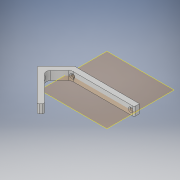
# Autodesk Inventor part: Part5
Saved by Autodesk Inventor 2019 (Build 230136000, 136)
## iProperties
Created: 2021-11-18
Part Number: Part5
Material: Generic
Document SubType Name: Modeling
Designer: Pokick
Density: 1 g/cm^3
Appearance: Default
Author: Pokick
Autodesk Inventor part; units mm, degrees
ref_plane "YZ Plane" through (0, 0, 0) normal (1, 0, 0) x (0, 1, 0)
ref_plane "XY Plane" through (0, 0, 0) normal (0, 0, 1) x (1, 0, 0)
sketch "Sketch1" plane through (0, 0, 0) normal (0, 0, 1) x (1, 0, 0)
  line L0 (-33, 45) -> (33, 45) construction
  line L1 (33, 45) -> (33, -45) construction
  line L2 (33, -45) -> (-33, -45) construction
  line L3 (-33, -45) -> (-33, 45) construction
  line L4 (-33, 45) -> (33, -45) construction
  line L5 (33, 45) -> (-33, -45) construction
  circle A0 centre (33, 45) radius 1.7
  circle A1 centre (-33, 45) radius 1.7
  point P0 (0, 0)
  dimension "d0" = 66
  dimension "d1" = 90
  dimension "d2" = 3.4
  dimension "d3" = 3.4
  constraints: 12 end point, 2 centre point, 2 coincident, 2 midpoint, 2 parallel, 1 horizontal, 1 perpendicular
  measures "d0" distance of L1.end L2.end
  measures "d1" distance of L0.end L1.end
  measures "d2" diameter of A0
  measures "d3" diameter of A1
ref_plane "Work Plane1" through (0, 45, 0) normal (0, 1, 0) x (-1, 0, 0)
sketch "Sketch2" plane through (0, 45, 0) normal (0, 1, 0) x (-1, 0, 0)
  line L0 (0, 0) -> (-37, 0)
  line L1 (0, 0) -> (37, 0)
  line L2 (37, 0) -> (58.2132, 21.2132)
  line L3 (58.2132, 21.2132) -> (-12.4975, 91.9239) construction
  line L4 (58.2132, 21.2132) -> (158.2132, 21.2132) construction
  line L5 (-37, 0) -> (21.2132, 58.2132) construction
  line L6 (-37, 0) -> (45.3259, 0) construction
  line L7 (21.2132, 58.2132) -> (58.2132, 21.2132)
  line L8 (37, 0) -> (37, 6) construction
  line L9 (43.7619, 6.7619) -> (39.5192, 11.0045) construction
  line L10 (43.7619, 6.7619) -> (49.7619, 6.7619) construction
  line L11 (34.5147, 6) -> (-31, 6)
  line L12 (-31, 6) -> (-37, 0) construction
  line L13 (39.5192, 11.0045) -> (34.5147, 6)
  line L14 (53.9706, 25.4558) -> (49.7279, 21.2132) construction
  line L15 (39.5192, 11.0045) -> (49.7279, 21.2132)
  line L16 (21.2132, 58.2132) -> (16.9706, 53.9706)
  line L17 (49.7279, 21.2132) -> (16.9706, 53.9706)
  line L18 (-37, 0) -> (-37, 6)
  line L19 (-37, 6) -> (-31, 6)
  dimension "d5" = 37
  dimension "d6" = 37
  dimension "d7" = 30
  dimension "d8" = 135
  dimension "d9" = 100
  dimension "d10" = 135
  dimension "d11" = 45
  dimension "d13" = 6
  dimension "d14" = 6
  dimension "d15" = 135
  dimension "d16" = 14.4513
  dimension "d17" = 6
  dimension "d18" = 20.1629
  dimension "d19" = 15.2132
  constraints: 40 end point, 6 horizontal, 5 point on line, 3 equal length, 3 perpendicular, 2 collinear, 2 vertical, 1 parallel
  measures "d5" distance of L0.start L0.end
  measures "d6" distance of L0.start L1.end
  measures "d7" distance of L1.end L2.end
  measures "d8" angle of L2 L1
  measures "d9" distance of L2.end L3.end
  measures "d10" angle of L4 L3
  measures "d11" angle of L6 L5
  measures "d13" distance of L1.end L8.end
  measures "d14" distance of L9.start L9.end
  measures "d15" angle of L10 L9
  measures "d16" distance between parallel lines of L10 L4
  measures "d17" distance of L14.start L14.end
  measures "d18" distance from line of L0.start L14
  measures "d19" distance between parallel lines of L11 L4
extrude "Extrusion1" add sketch "Sketch2" along normal mid plane 10
fillet "Fillet1" radius 5 2 edges at (-49.7279, 45, 21.2132) (-34.5147, 45, 6)
fillet "Fillet2" radius 0.5 1 edges at (37, 45, 0)
fillet "Fillet3" radius 2 1 edges at (-37, 45, 0)
fillet "Fillet4" radius 2 3 edges at (-58.2132, 45, 21.2132) (-16.9706, 45, 53.9706) (-21.2132, 45, 58.2132)
fillet "Fillet5" radius 2 1 edges at (37, 45, 6)
extrude "Extrusion2" cut sketch "Sketch1" along normal blind 10
sketch "Sketch3" plane through (-22.6274, 40, 56.799) normal (-0.7071068, 0, 0.7071068) x (0.7071068, 0, 0.7071068)
  line L0 (-39.3259, 0) -> (0, 0) construction
  line L1 (-48.3259, 0) -> (-48.3259, 10) construction
  line L2 (0, 0) -> (-48.3259, 0) construction
  line L3 (-48.3259, 0) -> (-48.3259, 10) construction
  line L4 (-48.3259, 10) -> (0, 10) construction
  line L5 (0, 10) -> (0, 0) construction
  line L6 (0, 0) -> (0, 10) projected
  line L7 (0, 5) -> (-48.6996, 5) construction
  ellipse E0 centre (-47.4975, 5) end of major axis (-47.4975, 3.3) minor radius 1.2021 projected
  line L8 (0, 5) -> (48.6996, 5) construction
  circle A0 centre (-24.3498, 5) radius 15 construction
  circle A1 centre (-9.3498, 5) radius 1.75
  circle A2 centre (-39.3498, 5) radius 1.75
  point P0 (-24.163, -40)
  dimension "d29" = 180
  dimension "d30" = 30
  dimension "d31" = 3.5
  dimension "d32" = 3.5
  constraints: 12 end point, 3 centre point, 2 horizontal, 2 midpoint, 2 parallel, 2 point on circle, 2 point on line, 1 collinear, 1 horizontal alignment, 1 perpendicular, 1 other
  measures "d29" angle of L7 L8
  measures "d30" diameter of A0
  measures "d31" diameter of A1
  measures "d32" diameter of A2
extrude "Extrusion3" cut sketch "Sketch3" against normal blind 10 contours A1 | A2
chamfer "Chamfer1" distance 1 angle 45 4 edges at (-26.2335, 45, 44.7076) (-45.3283, 46.229, 25.6128) (-45.3283, 43.771, 25.6128) (-47.2167, 45.0007, 23.2644)
chamfer "Chamfer2" distance 1 angle 45 4 edges at (-34.7, 44.9992, 6.5381) (-31.6151, 44.014, 6) (-31.6151, 45.986, 6) (31.3, 45, 6)
body "Solid1"
